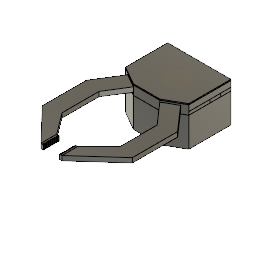
Prototype end effector (Autodesk Fusion 360 design; units mm, degrees)
Autodesk Fusion 360 part; units mm, degrees
note: some values were not read from the file. Set by a fixed rule: which sketch regions a step uses.
sketch "Sketch1" plane through (0, 0, 0) normal (0, 0, 1) x (1, 0, 0)
  line L0 (-5, 0) -> (45, 0)
  line L1 (45, 0) -> (80, 20)
  line L2 (80, 20) -> (80, 60)
  line L3 (-5, 0) -> (-40, 20)
  line L4 (-40, 20) -> (-40, 60)
  line L5 (-40, 60) -> (-40, 80)
  line L6 (-40, 80) -> (80, 80)
  line L7 (80, 80) -> (80, 60)
  line L8 (42, 70) -> (-3, 70)
  line L9 (19.5, 70) -> (19.5, 25)
  line L10 (-3, 47.5) -> (42, 47.5)
  circle A0 centre (19.5, 47.5) radius 20
  circle A1 centre (19.5, 47.5) radius 2.5
  line L11 (-5, 0) -> (-40, 20)
  circle A2 centre (-10, 25) radius 17.1272
  circle A3 centre (-10, 25) radius 2.5
  dimension "d2" = 5
  dimension "d3" = 5
  measures "d2" diameter of A1
  measures "d3" diameter of A3
extrude "Extrude1" add sketch "Sketch1" along normal blind 2 contours L0 L1 L2 L3 L4 L5 L6 L7 L11 | L9 L10 A0 A1 | L9 L10 A0 A1 | L9 L10 A1 | L9 L10 A1 | L9 L10 A0 A1 | L9 L10 A0 A1 A2 | L9 L10 A1 | L9 L10 A1 | A0 A2 | A0 A2 | A3 makes body 1
sketch "Sketch2" plane through (0, 0, 2) normal (0, 0, 1) x (-1, 0, 0)
  line L0 (-45, 0) -> (-80, -20)
  line L1 (-80, -20) -> (-80, -60)
  line L2 (-80, -60) -> (-80, -80)
  line L3 (-80, -80) -> (40, -80)
  line L4 (40, -80) -> (40, -20)
  line L5 (40, -20) -> (5, 0)
  line L6 (5, 0) -> (-45, 0)
  line L7 (40, -80) -> (-80, -80)
  line L8 (-80, -80) -> (-80, -20)
  line L9 (-80, -20) -> (-45, 0)
  line L10 (5, 0) -> (-45, 0)
  line L11 (5, 0) -> (40, -20)
  line L12 (40, -20) -> (40, -80)
  line L13 (0, -10) -> (-40, -10)
  line L14 (-40, -10) -> (-70, -25)
  line L15 (-70, -25) -> (-70, -70)
  line L16 (30, -70) -> (30, -25)
  line L17 (30, -25) -> (0, -10)
  line L18 (40, -80) -> (-80, -80)
  line L19 (-80, -80) -> (-80, -100)
  line L20 (-80, -100) -> (40, -100)
  line L21 (40, -100) -> (40, -80)
extrude "Extrude2" add sketch "Sketch2" against normal blind 2 contours L3 L7 L18 L19 L20 L21 bodies 1
sketch "Sketch3" plane through (0, 0, 2) normal (0, 0, 1) x (-1, 0, 0)
  line L0 (-45, 0) -> (-80, -20)
  line L1 (-80, -20) -> (-80, -60)
  line L2 (-80, -60) -> (-80, -80)
  line L3 (-80, -80) -> (-80, -100)
  line L4 (-80, -100) -> (40, -100)
  line L5 (40, -100) -> (40, -20)
  line L6 (40, -20) -> (5, 0)
  line L7 (5, 0) -> (-45, 0)
  line L8 (30, -90) -> (30, -30)
  line L9 (30, -30) -> (30, -25)
  line L10 (30, -25) -> (0, -10)
  line L11 (0, -10) -> (-40, -10)
  line L12 (-40, -10) -> (-70, -25)
  line L13 (-70, -25) -> (-70, -90)
  line L14 (-70, -90) -> (30, -90)
extrude "Extrude3" add sketch "Sketch3" along normal blind 3 bodies 1
sketch "Sketch4" plane through (0, 0, 2) normal (0, 0, 1) x (-1, 0, 0)
  line L0 (30, -90) -> (30, -25)
  line L1 (30, -25) -> (0, -10)
  line L2 (0, -10) -> (-40, -10)
  line L3 (-40, -10) -> (-70, -25)
  line L4 (-70, -25) -> (-70, -90)
  line L5 (-70, -90) -> (30, -90)
  line L6 (3.0542, -80) -> (-41.9458, -80)
  line L7 (-41.9458, -80) -> (-41.9458, -35)
  line L8 (-41.9458, -35) -> (3.0542, -35)
  line L9 (3.0542, -35) -> (3.0542, -80)
extrude "Extrude4" cut sketch "Sketch4" against normal blind 2 contours L6 L7 L8 L9 bodies 1
sketch "Sketch5" plane through (0, 0, 2) normal (0, 0, 1) x (-1, 0, 0)
  line L0 (-41.9458, -80) -> (-41.9458, -35)
  line L1 (-41.9458, -35) -> (3.0542, -35)
  line L2 (3.0542, -35) -> (3.0542, -80)
  line L3 (3.0542, -80) -> (-41.9458, -80)
  line L4 (30, -90) -> (30, -25)
  line L5 (30, -25) -> (0, -10)
  line L6 (0, -10) -> (-40, -10)
  line L7 (-40, -10) -> (-70, -25)
  line L8 (-70, -25) -> (-70, -90)
  line L9 (-70, -90) -> (30, -90)
  line L10 (3.0542, -35) -> (-41.9458, -80)
  line L11 (3.0542, -80) -> (-41.9458, -35)
  circle A0 centre (-19.4458, -57.5) radius 20.6234
extrude "Extrude5" add sketch "Sketch5" along normal blind 8 and the other way blind -5 separate body contours L10 L11 A0 | L10 L11 A0 | L10 L11 A0 | L10 L11 A0 makes body 2
sketch "Sketch6" plane through (4, 8, 0) normal (0.447214, 0.894427, 0) x (-0.894427, 0.447214, 0)
  line L0 (4.4721, 2) -> (38.0132, 2)
  line L1 (38.0132, 2) -> (38.0132, 5)
  line L2 (38.0132, 5) -> (4.4721, 5)
  line L3 (4.4721, 5) -> (4.4721, 2)
sketch "Sketch7" plane through (0, 0, 2) normal (0, 0, 1) x (-1, 0, 0)
  line L0 (-41.9458, -80) -> (-41.9458, -35)
  line L1 (-41.9458, -35) -> (3.0542, -35)
  line L2 (3.0542, -35) -> (3.0542, -80)
  line L3 (3.0542, -80) -> (-41.9458, -80)
  line L4 (30, -90) -> (30, -25)
  line L5 (30, -25) -> (0, -10)
  line L6 (0, -10) -> (-40, -10)
  line L7 (-40, -10) -> (-70, -25)
  line L8 (-70, -25) -> (-70, -90)
  line L9 (-70, -90) -> (30, -90)
  line L10 (-45, 0) -> (-80, -20)
  line L11 (30, -25) -> (0, -10)
  circle A0 centre (-0.7403, -26.7042) radius 15.2789
  circle A1 centre (-0.7403, -26.7042) radius 2.5
  dimension "d16" = 5
  measures "d16" diameter of A1
extrude "Extrude6" add sketch "Sketch7" along normal blind 8 contours A1 bodies 1
sketch "Sketch8" plane through (0, 0, 10) normal (0, 0, 1) x (-1, 0, 0)
  circle A0 centre (-0.7403, -26.7042) radius 2.5
  circle A1 centre (-0.7403, -26.7042) radius 15.401
extrude "Extrude7" add sketch "Sketch8" against normal blind 3 bodies 1
sketch "Sketch9" plane through (0, 0, 2) normal (0, 0, 1) x (-1, 0, 0)
  circle A0 centre (-0.7403, -26.7042) radius 2.5
  line L0 (-41.9458, -80) -> (-41.9458, -35)
  line L1 (-41.9458, -35) -> (3.0542, -35)
  line L2 (3.0542, -35) -> (3.0542, -80)
  line L3 (3.0542, -80) -> (-41.9458, -80)
  line L4 (30, -90) -> (30, -25)
  line L5 (30, -25) -> (0, -10)
  line L6 (0, -10) -> (-40, -10)
  line L7 (-40, -10) -> (-70, -25)
  line L8 (-70, -25) -> (-70, -90)
  line L9 (-70, -90) -> (30, -90)
  circle A1 centre (-48.0475, -30.1202) radius 14.061
  circle A2 centre (-48.0475, -30.1202) radius 2.5
  dimension "d21" = 5
  measures "d21" diameter of A2
extrude "Extrude8" add sketch "Sketch9" along normal blind 10 contours A2 bodies 1
sketch "Sketch10" plane through (0, 0, 12) normal (0, 0, 1) x (-1, 0, 0)
  circle A0 centre (-48.0475, -30.1202) radius 2.5
sketch "Sketch11" plane through (0, 0, 2) normal (0, 0, 1) x (-1, 0, 0)
  circle A0 centre (-48.0475, -30.1202) radius 2.5
  circle A1 centre (-0.7403, -26.7042) radius 2.5
  line L0 (-41.9458, -80) -> (-41.9458, -35)
  line L1 (-41.9458, -35) -> (3.0542, -35)
  line L2 (3.0542, -35) -> (3.0542, -80)
  line L3 (3.0542, -80) -> (-41.9458, -80)
  line L4 (30, -90) -> (30, -25)
  line L5 (30, -25) -> (0, -10)
  line L6 (0, -10) -> (-40, -10)
  line L7 (-40, -10) -> (-70, -25)
  line L8 (-70, -25) -> (-70, -90)
  line L9 (-70, -90) -> (30, -90)
  circle A2 centre (-48.0475, -30.1202) radius 14.3971
extrude "Extrude9" add sketch "Sketch11" along normal blind 8 and the other way blind -5 contours L0 L1 A2 | L0 L1 A2 bodies 1
sketch "Sketch12" plane through (0, 0, 2) normal (0, 0, 1) x (-1, 0, 0)
  circle A0 centre (-48.0475, -30.1202) radius 2.5
  circle A1 centre (-0.7403, -26.7042) radius 2.5
  line L0 (-41.9458, -80) -> (-41.9458, -35)
  line L1 (-41.9458, -35) -> (3.0542, -35)
  line L2 (3.0542, -35) -> (3.0542, -80)
  line L3 (3.0542, -80) -> (-41.9458, -80)
  line L4 (30, -90) -> (30, -25)
  line L5 (30, -25) -> (0, -10)
  line L6 (0, -10) -> (-40, -10)
  line L7 (-40, -10) -> (-70, -25)
  line L8 (-70, -25) -> (-70, -90)
  line L9 (-70, -90) -> (30, -90)
  circle A2 centre (-48.0475, -30.1202) radius 14.3971
  circle A3 centre (-19.4458, -57.5) radius 20.6234
  circle A4 centre (-46, -51) radius 6.7759
  circle A5 centre (-46, -51) radius 2.5
  dimension "d28" = 5
  measures "d28" diameter of A5
extrude "Extrude10" add sketch "Sketch12" along normal blind 10 contours A5 bodies 1
sketch "Sketch13" plane through (0, 0, 2) normal (0, 0, 1) x (-1, 0, 0)
  circle A0 centre (-46, -51) radius 2.5
  circle A1 centre (-48.0475, -30.1202) radius 2.5
  circle A2 centre (-0.7403, -26.7042) radius 2.5
  line L0 (-41.9458, -80) -> (-41.9458, -35)
  line L1 (-41.9458, -35) -> (3.0542, -35)
  line L2 (3.0542, -35) -> (3.0542, -80)
  line L3 (3.0542, -80) -> (-41.9458, -80)
  line L4 (30, -90) -> (30, -25)
  line L5 (30, -25) -> (0, -10)
  line L6 (0, -10) -> (-40, -10)
  line L7 (-40, -10) -> (-70, -25)
  line L8 (-70, -25) -> (-70, -90)
  line L9 (-70, -90) -> (30, -90)
  circle A3 centre (-46, -51) radius 6.5162
extrude "Extrude11" add sketch "Sketch13" along normal blind 8 and the other way blind -5 contours L0 A3 | L0 A3 bodies 1
extrude "Extrude12" add 1 faces at (3.3333, 96.6667, 5) along direction (0, 0, 1) blind 1 on bodies 1 bodies 1
sketch "Sketch14" plane through (0, 0, 6) normal (0, 0, 1) x (-1, 0, 0)
  line L0 (30, -90) -> (-70, -90)
  line L1 (-70, -90) -> (-70, -25)
  line L2 (-70, -25) -> (-40, -10)
  line L3 (-40, -10) -> (0, -10)
  line L4 (0, -10) -> (30, -25)
  line L5 (30, -25) -> (30, -90)
  line L6 (5, 0) -> (-45, 0)
  line L7 (-45, 0) -> (-80, -20)
  line L8 (-80, -20) -> (-80, -60)
  line L9 (-80, -60) -> (-80, -80)
  line L10 (-80, -80) -> (-80, -100)
  line L11 (-80, -100) -> (40, -100)
  line L12 (40, -100) -> (40, -20)
  line L13 (40, -20) -> (5, 0)
  line L14 (30, -25) -> (30.5223, -14.5842)
  line L15 (30.5223, -14.5842) -> (40, -20)
  line L16 (40, -20) -> (40, -100)
  line L17 (40, -100) -> (-80, -100)
  line L18 (-80, -20) -> (-80, -100)
  line L19 (-70, -25) -> (-70, -14.2857)
  line L20 (-70, -14.2857) -> (-80, -20)
  line L21 (-70, -25) -> (-70, -90)
  line L22 (-70, -90) -> (30, -90)
  line L23 (30, -90) -> (30, -25)
  line L24 (2.7926, 0) -> (0, -10)
  line L25 (-40, -10) -> (-45, 0)
extrude "Extrude13" add sketch "Sketch14" along normal blind 8 contours L0 L1 L5 L7 L8 L9 L10 L11 L12 L13 L14 L15 L16 L17 L18 L19 L20 L21 L22 L23 bodies 1
sketch "Sketch15" plane through (0, 0, 0) normal (0, 1, 0) x (1, 0, 0)
sketch "Sketch16" plane through (0, 0, 6) normal (0, 0, 1) x (-1, 0, 0)
  line L0 (30, -25) -> (30.5223, -14.5842)
  line L1 (30.5223, -14.5842) -> (5, 0)
  line L2 (5, 0) -> (-45, 0)
  line L3 (-45, 0) -> (-70, -14.2857)
  line L4 (-70, -14.2857) -> (-70, -25)
  line L5 (-70, -25) -> (-40, -10)
  line L6 (-40, -10) -> (0, -10)
  line L7 (0, -10) -> (30, -25)
  line L8 (5, 0) -> (0, -10)
  line L9 (-40, -10) -> (-45, 0)
extrude "Extrude14" add sketch "Sketch16" along normal blind 8 contours L2 L6 L8 L9 bodies 1
sketch "Sketch17" plane through (0, 0, 10) normal (0, 0, 1) x (-1, 0, 0)
  circle A0 centre (-0.7403, -26.7042) radius 15.401
  circle A1 centre (-0.7403, -26.7042) radius 2.5
  dimension "d41" = 5
  measures "d41" diameter of A1
extrude "Extrude15" add sketch "Sketch17" along normal blind 2 contours A1 bodies 1
sketch "Sketch18" plane through (0, 0, 10) normal (0, 0, 1) x (-1, 0, 0)
  circle A0 centre (-19.4458, -57.5) radius 20.6234
  circle A1 centre (-19.4458, -57.5) radius 2.5
  dimension "d44" = 5
  measures "d44" diameter of A1
extrude "Extrude16" add sketch "Sketch18" along normal blind 2 contours A1 bodies 2
sketch "Sketch19" plane through (0, 0, 0) normal (0, 0, 1) x (1, 0, 0)
  line L0 (-5, 0) -> (-30, -40)
  line L1 (-30, -40) -> (-30, -110)
  line L2 (-30, -110) -> (0, -150)
  line L3 (-30.5223, 14.5842) -> (-60.4542, -33.3068)
  line L4 (-60.4542, -33.3068) -> (-60.4542, -117.2129)
  line L5 (-60.4542, -117.2129) -> (0, -180)
  line L6 (0, -180) -> (0, -150)
  line L7 (-30.5223, 14.5842) -> (-5, 0)
extrude "Extrude17" add sketch "Sketch19" along normal blind 14 and the other way blind -5 separate body makes body 3
sketch "Sketch20" plane through (0, 0, 0) normal (0, 0, 1) x (1, 0, 0)
  line L0 (45, 0) -> (80, -40)
  line L1 (45, 0) -> (80, 20)
  line L2 (45, 0) -> (70, 14.2857)
  line L3 (70, 14.2857) -> (110.1239, -31.5701)
  line L4 (110.1239, -31.5701) -> (110.1239, -116.9355)
  line L5 (-60.4542, -33.3068) -> (-60.4542, -117.2129)
  line L6 (80, -40) -> (80, -110)
  line L7 (80, -110) -> (40, -150)
  line L8 (40, -150) -> (40, -180)
  line L9 (40, -180) -> (110.1239, -116.9355)
extrude "Extrude18" add sketch "Sketch20" along normal blind 14 and the other way blind -5 separate body makes body 4
sketch "Sketch21" plane through (0, 0, 0) normal (0, 0, 1) x (1, 0, 0)
extrude "Extrude19" add 1 faces at (-0.056, 26.4586, 12) along direction (0, 0, 1) blind 2 on bodies 1 bodies 1
extrude "Extrude20" add 1 faces at (18.6494, 57.9775, 12) along direction (0, 0, 1) blind 2 on bodies 2 bodies 2
extrude "Extrude21" add 1 faces at (45.3392, 50.652, 12) along direction (0, 0, 1) blind 2 on bodies 1 bodies 1
extrude "Extrude22" add sketch "Sketch10" along normal blind 2 bodies 1
sketch "Sketch22" plane through (0, 0, 7) normal (0, 0, -1) x (1, 0, 0)
  circle A0 centre (19.4458, -57.5) radius 20.6234
  circle A1 centre (19.4458, -57.5) radius 2.5
extrude "Extrude23" add sketch "Sketch22" along normal blind 5 contours A1 bodies 2
sketch "Sketch23" plane through (0, 0, 10) normal (0, 0, 1) x (-1, 0, 0)
  circle A0 centre (-19.4458, -57.5) radius 2.5
  circle A1 centre (-19.4458, -57.5) radius 20.6234
sketch "Sketch24" plane through (0, 0, 0) normal (0, 1, 0) x (1, 0, 0)
extrude "Extrude24" add 1 faces at (20.1966, 57.8616, 2) along direction (0, 0, -1) blind 8 on bodies 2 bodies 2
sketch "Sketch25" plane through (0, 0, 0) normal (0, 1, 0) x (1, 0, 0)
sketch "Sketch26" plane through (0, 0, 14) normal (0, 0, 1) x (-1, 0, 0)
  line L0 (-70, -90) -> (-70, -14.2857)
  line L1 (-70, -14.2857) -> (-80, -20)
  line L2 (-80, -20) -> (-80, -100)
  line L3 (-80, -100) -> (40, -100)
  line L4 (40, -100) -> (40, -20)
  line L5 (40, -20) -> (30.5223, -14.5842)
  line L6 (30.5223, -14.5842) -> (30, -25)
  line L7 (30, -25) -> (30, -90)
  line L8 (30, -90) -> (-70, -90)
  line L9 (5, 0) -> (40, -20)
  line L10 (40, -20) -> (40, -100)
  line L11 (40, -100) -> (-80, -100)
  line L12 (-80, -100) -> (-80, -20)
  line L13 (-80, -20) -> (-45, 0)
  line L14 (-45, 0) -> (5, 0)
  line L15 (0, -10) -> (30, -25)
  line L16 (30, -25) -> (30, -90)
  line L17 (30, -90) -> (-70, -90)
  line L18 (-70, -90) -> (-70, -25)
  line L19 (-40, -10) -> (-70, -25)
  line L20 (-70, -25) -> (-40, -10)
  line L21 (-40, -10) -> (0, -10)
extrude "Extrude25" add sketch "Sketch26" along normal blind 3 contours L0 L1 L2 L3 L4 L5 L6 L7 L8 L9 L10 L11 L12 L13 L16 L17 L18 | L0 L6 L9 L13 L14 L15 L19 L20 L21 bodies 1 3 4
move_face "MoveFace1" by (0, 30, 0) 1 faces at (-27.6847, 66.6667, 0) on bodies 1
sketch "Sketch27" plane through (0, 0, 17) normal (0, 0, 1) x (-1, 0, 0)
  line L0 (-70, -25) -> (-40, -10)
  line L1 (-40, -10) -> (0, -10)
  line L2 (0, -10) -> (30, -25)
  line L3 (30, -25) -> (30, -90)
  line L4 (30, -90) -> (-70, -90)
  line L5 (-70, -90) -> (-70, -25)
  line L6 (-45, 0) -> (-80, -20)
  line L7 (-80, -20) -> (-80, -100)
  line L8 (-80, -100) -> (40, -100)
  line L9 (40, -100) -> (40, -20)
  line L10 (40, -20) -> (5, 0)
  line L11 (5, 0) -> (-45, 0)
  line L12 (40, -100) -> (40, -20)
  line L13 (40, -20) -> (5, 0)
  line L14 (5, 0) -> (-45, 0)
  line L15 (-45, 0) -> (-80, -20)
  line L16 (-80, -20) -> (-80, -100)
  line L17 (40, -100) -> (-80, -100)
extrude "Extrude26" add sketch "Sketch27" along normal blind 2 separate body contours L0 L1 L2 L3 L4 L5 | L6 L7 L8 L9 L10 L11 L12 L13 L14 L15 L16 L17 makes body 5
sketch "Sketch28" plane through (0, 0, -6) normal (0, 0, -1) x (1, 0, 0)
  circle A0 centre (19.4458, -57.5) radius 2.5
  line L0 (-1.8129, -35.867) -> (41.1871, -35.867)
  line L1 (41.1871, -35.867) -> (41.1871, -78.867)
  line L2 (41.1871, -78.867) -> (-1.8129, -78.867)
  line L3 (-1.8129, -78.867) -> (-1.8129, -35.867)
  dimension "d71" = 43
  dimension "d72" = 43
  measures "d71" distance of origin
extrude "Extrude27" add sketch "Sketch28" along normal blind 48 separate body makes body 6
extrude "Extrude28" add 1 faces at (20.1966, 57.8616, -6) along direction (0, 0, -1) blind 48 on bodies 2 bodies 2 6
sketch "Sketch29" plane through (0, 0, 0) normal (0, 0, -1) x (1, 0, 0)
  line L0 (41.9458, -35) -> (41.9458, -80)
  line L1 (41.9458, -80) -> (-3.0542, -80)
  line L2 (-3.0542, -80) -> (-3.0542, -35)
  line L3 (-3.0542, -35) -> (41.9458, -35)
  line L4 (80, -20) -> (45, 0)
  line L5 (45, 0) -> (-5, 0)
  line L6 (-5, 0) -> (-40, -20)
  line L7 (-40, -20) -> (-40, -100)
  line L8 (-40, -100) -> (80, -100)
  line L9 (80, -100) -> (80, -80)
  line L10 (80, -80) -> (80, -60)
  line L11 (80, -60) -> (80, -20)
  line L12 (-40, -20) -> (-5, 0)
  line L13 (-5, 0) -> (45, 0)
  line L14 (80, -20) -> (45, 0)
  line L15 (80, -20) -> (80, -100)
  line L16 (80, -100) -> (-40, -100)
  line L17 (-40, -100) -> (-40, -20)
  line L18 (-30, -90) -> (70, -90)
  line L19 (25.2705, -80) -> (25.2705, -90)
  line L20 (15, -90) -> (15, -80)
  line L21 (15, -90) -> (-30, -90)
  line L22 (-30, -25) -> (-30, -90)
  line L23 (-30, -90) -> (-30, -65)
  line L24 (-3.0542, -65.1427) -> (-30, -65)
  line L25 (-30, -55) -> (-3.0542, -54.8201)
  line L26 (-30, -55) -> (-30, -25)
  line L27 (-3.0542, -65.1427) -> (-3.0542, -54.8201)
  line L28 (-3.0542, -65.1427) -> (-3.0542, -54.8201)
  line L29 (15, -80) -> (25.2705, -80)
  line L30 (-30, -25) -> (0, -10)
  line L31 (-30, -25) -> (0, -10)
  line L32 (40, -10) -> (0, -10)
  line L33 (20, -33.5494) -> (20, -35)
  line L34 (15, -35) -> (15, -10)
  line L35 (15, -10) -> (0, -10)
  line L36 (25, -35) -> (25, -10)
  line L37 (25, -35) -> (15, -35)
  line L38 (25, -10) -> (40, -10)
  line L39 (70, -90) -> (70, -25)
  line L40 (70, -25) -> (40, -10)
  line L41 (70, -90) -> (25.2705, -90)
  line L42 (70, -65) -> (41.9458, -65)
  line L43 (41.9458, -65) -> (41.9458, -55)
  line L44 (41.9458, -55) -> (70, -55)
extrude "Extrude29" add sketch "Sketch29" along normal blind 54 separate body contours L0 L39 L42 L43 L44 | L3 L32 L34 L36 L37 | L1 L18 L19 L20 L29 | L2 L22 L24 L25 L27 L28 | L4 L5 L6 L7 L8 L9 L10 L11 L12 L13 L14 L15 L16 L17 makes body 7
sketch "Sketch30" plane through (0, 100, 0) normal (0, 1, 0) x (-1, 0, 0)
  line L0 (40, 0) -> (-80, 0)
  line L1 (-80, 0) -> (-80, -54)
  line L2 (-80, -54) -> (40, -54)
  line L3 (40, -54) -> (40, 0)
  line L4 (-80, 19) -> (40, -54)
  line L5 (40, 19) -> (-80, -54)
  circle A0 centre (-20, -17.5) radius 2.5
  dimension "d79" = 5
  measures "d79" diameter of A0
extrude "Extrude30" cut sketch "Sketch30" against normal blind 20 contours L4 L5 A0 | L4 L5 A0 | L4 L5 A0 | L4 L5 A0 bodies 7
sketch "Sketch31" plane through (0, 0, -54) normal (0, 0, -1) x (1, 0, 0)
  line L0 (70, -65) -> (70, -90)
  line L1 (70, -90) -> (25.2705, -90)
  line L2 (25.2705, -90) -> (25.2705, -80)
  line L3 (25.2705, -80) -> (15, -80)
  line L4 (15, -80) -> (15, -90)
  line L5 (15, -90) -> (-30, -90)
  line L6 (-30, -90) -> (-30, -65)
  line L7 (-30, -65) -> (-3.0542, -65.1427)
  line L8 (-3.0542, -65.1427) -> (-3.0542, -54.8201)
  line L9 (-3.0542, -54.8201) -> (-30, -55)
  line L10 (-30, -55) -> (-30, -25)
  line L11 (-30, -25) -> (0, -10)
  line L12 (0, -10) -> (15, -10)
  line L13 (15, -10) -> (15, -35)
  line L14 (15, -35) -> (25, -35)
  line L15 (25, -35) -> (25, -10)
  line L16 (25, -10) -> (40, -10)
  line L17 (40, -10) -> (70, -25)
  line L18 (70, -25) -> (70, -55)
  line L19 (70, -55) -> (41.9458, -55)
  line L20 (41.9458, -55) -> (41.9458, -65)
  line L21 (41.9458, -65) -> (70, -65)
  line L22 (80, -20) -> (45, 0)
  line L23 (45, 0) -> (-5, 0)
  line L24 (-5, 0) -> (-40, -20)
  line L25 (-40, -20) -> (-40, -100)
  line L26 (-40, -100) -> (80, -100)
  line L27 (80, -100) -> (80, -20)
  line L28 (45, 0) -> (80, -20)
  line L29 (45, 0) -> (-5, 0)
  line L30 (-5, 0) -> (-40, -20)
  line L31 (-40, -20) -> (-40, -100)
  line L32 (-40, -100) -> (80, -100)
  line L33 (80, -100) -> (80, -20)
extrude "Extrude31" add sketch "Sketch31" along normal blind 2 contours L0 L1 L2 L3 L4 L5 L6 L7 L8 L9 L10 L11 L12 L13 L14 L15 L16 L17 L18 L19 L20 L21 | L22 L23 L24 L25 L26 L27 L28 L29 L30 L31 L32 L33 bodies 2 7
sketch "Sketch32" plane through (0, 0, 5) normal (0, 0, -1) x (1, 0, 0)
  line L0 (80, 40) -> (45, 0)
  line L1 (45, 0) -> (70, -14.2857)
  line L2 (70, -14.2857) -> (110.1239, 31.5701)
  line L3 (110.1239, 31.5701) -> (110.1239, 116.9355)
  line L4 (110.1239, 116.9355) -> (40, 180)
  line L5 (40, 180) -> (40, 150)
  line L6 (40, 150) -> (80, 110)
  line L7 (80, 110) -> (80, 40)
  line L8 (40, 150) -> (35, 150)
  line L9 (35, 150) -> (35, 152)
  line L10 (35, 152) -> (37, 152)
  line L11 (37, 152) -> (37, 154)
  line L12 (37, 154) -> (35, 154)
  line L13 (35, 154) -> (35, 156)
  line L14 (35, 156) -> (37, 156)
  line L15 (37, 156) -> (37, 158)
  line L16 (37, 158) -> (35, 158)
  line L17 (35, 158) -> (35, 160)
  line L18 (35, 160) -> (37, 160)
  line L19 (37, 160) -> (37, 162)
  line L20 (37, 162) -> (35, 162)
  line L21 (35, 162) -> (35, 164)
  line L22 (35, 164) -> (37, 164)
  line L23 (37, 164) -> (37, 166)
  line L24 (37, 166) -> (35, 166)
  line L25 (35, 166) -> (35, 168)
  line L26 (35, 168) -> (37, 168)
  line L27 (37, 168) -> (37, 170)
  line L28 (37, 170) -> (35, 170)
  line L29 (35, 170) -> (35, 172)
  line L30 (35, 172) -> (37, 172)
  line L31 (37, 172) -> (37, 174)
  line L32 (37, 174) -> (35, 174)
  line L33 (35, 174) -> (35, 176)
  line L34 (35, 176) -> (37, 176)
  line L35 (37, 176) -> (37, 177.5482)
  line L36 (37, 177.5482) -> (35, 177.5482)
  line L37 (35, 177.5482) -> (35, 180)
  line L38 (35, 180) -> (40, 180)
  dimension "d84" = 2
extrude "Extrude32" add sketch "Sketch32" against normal blind 9 separate body contours L5 L8 L9 L10 L11 L12 L13 L14 L15 L16 L17 L18 L19 L20 L21 L22 L23 L24 L25 L26 L27 L28 L29 L30 L31 L32 L33 L34 L35 L36 L37 L38 makes body 8
sketch "Sketch33" plane through (0, 0, 14) normal (0, 0, 1) x (-1, 0, 0)
  line L0 (60.4542, 33.3068) -> (60.4542, 117.2129)
  line L1 (60.4542, 117.2129) -> (0, 180)
  line L2 (0, 180) -> (0, 150)
  line L3 (0, 150) -> (30, 110)
  line L4 (30, 110) -> (30, 40)
  line L5 (30, 40) -> (5, 0)
  line L6 (5, 0) -> (30.5223, -14.5842)
  line L7 (30.5223, -14.5842) -> (60.4542, 33.3068)
  line L8 (0, 150) -> (-5, 150)
  line L9 (-5, 150) -> (-5, 152)
  line L10 (-5, 152) -> (-3, 152)
  line L11 (-3, 152) -> (-3, 154)
  line L12 (-3, 154) -> (-5, 154)
  line L13 (-5, 154) -> (-5, 156)
  line L14 (-5, 156) -> (-3, 156)
  line L15 (-3, 156) -> (-3, 158)
  line L16 (-3, 158) -> (-5, 158)
  line L17 (-5, 158) -> (-5, 160)
  line L18 (-5, 160) -> (-4, 160)
  line L19 (-4, 160) -> (-3, 160)
  line L20 (-3, 160) -> (-3, 162)
  line L21 (-3, 162) -> (-5, 162)
  line L22 (-5, 162) -> (-5, 164)
  line L23 (-5, 164) -> (-3, 164)
  line L24 (-3, 164) -> (-3, 166)
  line L25 (-3, 166) -> (-5, 166)
  line L26 (-5, 166) -> (-5, 168)
  line L27 (-5, 168) -> (-3, 168)
  line L28 (-3, 168) -> (-3, 170)
  line L29 (-3, 170) -> (-5, 170)
  line L30 (-5, 170) -> (-5, 172)
  line L31 (-5, 172) -> (-3, 172)
  line L32 (-3, 172) -> (-3, 174)
  line L33 (-3, 174) -> (-5, 174)
  line L34 (-5, 174) -> (-5, 176)
  line L35 (-5, 176) -> (-3, 176)
  line L36 (-3, 176) -> (-3, 178)
  line L37 (-3, 178) -> (-5, 178)
  line L38 (-5, 178) -> (-5, 180)
  line L39 (-5, 180) -> (0, 180)
extrude "Extrude33" add sketch "Sketch33" against normal blind 9 separate body contours L2 L8 L9 L10 L11 L12 L13 L14 L15 L16 L17 L18 L19 L20 L21 L22 L23 L24 L25 L26 L27 L28 L29 L30 L31 L32 L33 L34 L35 L36 L37 L38 L39 makes body 9
